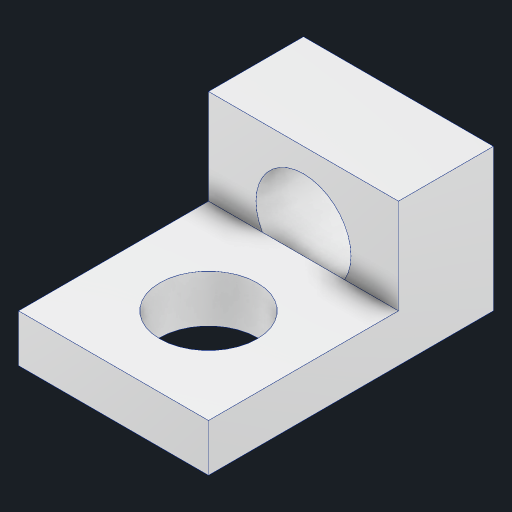
# Autodesk Inventor part: OUTK_022_BadPivot
Saved by Autodesk Inventor 2024.2 (Build 282272000, 272)
## iProperties
Created: 2024-12-08
Part Number: OUTK_022_BadPivot
Material: Aluminum 6061
Document SubType Name: Modeling
Designer: Bryan
Density: 2.7 g/cm^3
Appearance: Aluminum - Flat
Author: Bryan
Autodesk Inventor part; units mm, degrees
ref_plane "YZ Plane" through (0, 0, 0) normal (1, 0, 0) x (0, 1, 0)
ref_plane "XZ Plane" through (0, 0, 0) normal (0, 1, 0) x (-1, 0, 0)
ref_plane "XY Plane" through (0, 0, 0) normal (0, 0, 1) x (1, 0, 0)
sketch "Sketch1" plane through (0, 0, 0) normal (0, 1, 0) x (-1, 0, 0)
  circle A0 centre (0, 0) radius 3.2512
  line L0 (6.35, 6.35) -> (-6.35, 6.35)
  line L1 (-6.35, 6.35) -> (-6.35, -12.7)
  line L2 (-6.35, -12.7) -> (6.35, -12.7)
  line L3 (6.35, -12.7) -> (6.35, 6.35)
  point P0 (0, 6.35)
  dimension "d0" = 6.5024
  dimension "d1" = 12.7
  dimension "d2" = 19.05
  dimension "d3" = 6.35
  constraints: 8 end point, 2 parallel, 1 centre point, 1 coincident, 1 horizontal, 1 midpoint, 1 perpendicular, 1 vertical alignment
  measures "d0" diameter of A0
  measures "d1" distance of L2.end L1.end
  measures "d2" distance of L1.end L0.end
  measures "d3" distance from line of L0 point (0, 0)
extrude "Extrusion1" add sketch "Sketch1" along normal blind 3.175
sketch "Sketch2" plane through (0, 3.175, 0) normal (0, 1, 0) x (1, 0, 0)
  line L0 (6.35, 12.7) -> (-6.35, 12.7) projected
  line L1 (6.35, -6.35) -> (6.35, 12.7) projected
  line L2 (-6.35, 12.7) -> (6.35, 12.7)
  line L3 (6.35, 12.7) -> (6.35, 6.35)
  line L4 (6.35, 6.35) -> (-6.35, 6.35)
  line L5 (-6.35, 6.35) -> (-6.35, 12.7)
  point P0 (0, 0)
  dimension "d6" = 6.35
  constraints: 8 end point, 2 parallel, 1 horizontal, 1 perpendicular, 1 point on line
  measures "d6" distance of L2.end L3.end
extrude "Extrusion2" add sketch "Sketch2" along normal blind 6.35
sketch "Sketch3" plane through (6.35, 0, -12.7) normal (0, 0, -1) x (-1, 0, 0)
  circle A0 centre (6.35, 4.7625) radius 3.175
  line L0 (12.7, 0) -> (12.7, 9.525) projected
  line L1 (0, 9.525) -> (12.7, 9.525) projected
  point P0 (6.35, 0)
  point P1 (12.7, 4.7625)
  point P2 (6.35, 9.525)
  dimension "d9" = 6.35
  constraints: 2 midpoint, 1 centre point, 1 horizontal alignment, 1 vertical alignment
  measures "d9" diameter of A0
extrude "Extrusion3" cut sketch "Sketch3" against normal up to surface (6.35 mm away)
body "Solid1"
